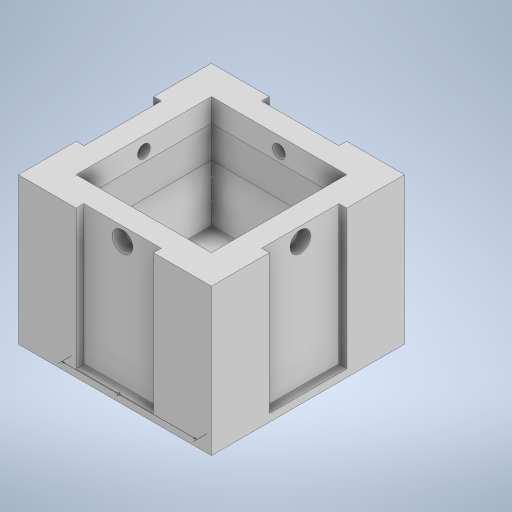
# Autodesk Inventor part: Ulepszona wersja
Saved by Autodesk Inventor 2024 (Build 280153000, 153)
## iProperties
Created: 2023-11-08
Part Number: Ulepszona wersja
Material: Generic
Document SubType Name: Modeling
Designer: Piotrek
Density: 1 g/cm^3
Appearance: Default
Author: Piotrek
Autodesk Inventor part; units mm, degrees
ref_plane "YZ Plane" through (0, 0, 0) normal (1, 0, 0) x (0, 1, 0)
ref_plane "XZ Plane" through (0, 0, 0) normal (0, 1, 0) x (-1, 0, 0)
sketch "Sketch1" plane through (0, 0, 0) normal (0, 1, 0) x (-1, 0, 0)
  line L0 (25, 25) -> (-25, 25)
  line L1 (-25, 25) -> (-25, -25)
  line L2 (-25, -25) -> (25, -25)
  line L3 (25, -25) -> (25, 25)
  line L4 (25, 25) -> (-25, -25) construction
  line L5 (-25, 25) -> (25, -25) construction
  line L6 (-22.5, 22.5) -> (22.5, 22.5)
  line L7 (22.5, 22.5) -> (22.5, -22.5)
  line L8 (22.5, -22.5) -> (-22.5, -22.5)
  line L9 (-22.5, -22.5) -> (-22.5, 22.5)
  line L10 (-22.5, 22.5) -> (22.5, -22.5) construction
  line L11 (22.5, 22.5) -> (-22.5, -22.5) construction
  point P0 (0, 0)
  dimension "d0" = 50
  dimension "d1" = 50
  dimension "d2" = 45
  dimension "d3" = 45
  constraints: 24 end point, 4 midpoint, 4 parallel, 2 horizontal, 2 perpendicular
  measures "d0" distance of L2.end L1.end
  measures "d1" distance of L1.end L0.end
  measures "d2" distance of L7.end L8.end
  measures "d3" distance of L6.end L7.end
extrude "Extrusion1" add sketch "Sketch1" along normal blind 30
extrude "Extrusion2" add sketch "Sketch1" along normal blind 2 contours L6 L7 L8 L9
sketch "Sketch2" plane through (0, 30, 0) normal (0, 1, 0) x (1, 0, 0)
  point P0 (0, 0)
sketch "Sketch3" plane through (0, 30, 0) normal (0, 1, 0) x (1, 0, 0)
  line L0 (17.5, -17.5) -> (-17.5, -17.5)
  line L1 (-17.5, -17.5) -> (-17.5, 17.5)
  line L2 (-17.5, 17.5) -> (17.5, 17.5)
  line L3 (17.5, 17.5) -> (17.5, -17.5)
  line L4 (17.5, -17.5) -> (-17.5, 17.5) construction
  line L5 (-17.5, -17.5) -> (17.5, 17.5) construction
  line L6 (-25, 25) -> (-25, -25) projected
  line L7 (25, -25) -> (-25, -25)
  line L8 (-25, -25) -> (-25, 25)
  line L9 (-25, 25) -> (25, 25)
  line L10 (25, 25) -> (25, -25)
  line L11 (25, -25) -> (-25, 25) construction
  line L12 (-25, -25) -> (25, 25) construction
  point P0 (0, 0)
  dimension "d8" = 35
  dimension "d9" = 35
  constraints: 24 end point, 4 midpoint, 4 parallel, 2 horizontal, 2 perpendicular
  measures "d8" distance of L1.end L2.end
  measures "d9" distance of L0.end L1.end
extrude "Extrusion3" add sketch "Sketch3" along normal blind 5.5
ref_plane "Work Plane1" through (0, 17.75, 0) normal (0, 1, 0) x (1, 0, 0)
chamfer "Chamfer1" distance 5 distance2 13.25 4 edges at (22.5, 30, 0) (0, 30, -22.5) (-22.5, 30, 0) (0, 30, 22.5) measured on face at (-5.8333, 30, 20.8333)
sketch "Sketch5" plane through (0, 35.5, 0) normal (0, 1, 0) x (1, 0, 0)
  point P0 (0, 0)
sketch "Sketch6" plane through (-17.5, 35.5, -17.5) normal (0, 0, 1) x (1, 0, 0)
  circle A0 centre (17.5, -3) radius 1.5
  line L0 (0, 0) -> (35, 0) projected
  point P0 (17.5, -35.5)
  point P1 (17.5, 0)
  dimension "d21" = 3
  dimension "d30" = 3
  constraints: 1 centre point, 1 midpoint
  measures "d21" diameter of A0
  measures "d30" distance of A0.centre point (17.5, 0)
extrude "Extrusion5" cut sketch "Sketch6" against normal through all
sketch "Sketch7" plane through (0, 35.5, 0) normal (0, 1, 0) x (1, 0, 0)
  line L0 (25, 25) -> (-25, 25) projected
  line L1 (10, 25) -> (0, 25)
  line L2 (10, 25) -> (-10, 25)
  line L3 (-10, 25) -> (10, 25)
  line L4 (10, 25) -> (10, 23)
  line L5 (10, 23) -> (-10, 23)
  line L6 (-10, 23) -> (-10, 25)
  point P0 (0, 0)
  dimension "d24" = 20
  dimension "d25" = 2
  constraints: 12 end point, 2 parallel, 2 point on line, 1 horizontal, 1 midpoint, 1 perpendicular
  measures "d24" distance of L1.start L2.end
  measures "d25" distance of L3.end L4.end
extrude "Extrusion6" cut sketch "Sketch7" against normal through all
sketch "Sketch9" plane through (10, 35.5, -23) normal (0, 0, -1) x (-1, 0, 0)
  circle A0 centre (10, -3) radius 1.5 projected
  circle A1 centre (10, -3) radius 2.5
  point P0 (10, -35.5)
  dimension "d37" = 3
  constraints: 1 centre point, 1 coincident
  measures "d37" diameter of A0
extrude "Extrusion7" cut sketch "Sketch9" against normal blind 3
pattern_circular "Circular Pattern2" count 4 over 360 about axis through (0, -10, 0) along (0, 1, 0) of "Extrusion7", "Extrusion6", "Extrusion5"
sketch "Sketch11" plane through (0, 32.5, -20) normal (0, 0, -1) x (-1, 0, 0)
  circle A0 centre (0, 0) radius 1.65
  circle A1 centre (0, 0) radius 2.65
  point P0 (0, -32.5)
  dimension "d38" = 3.3
  dimension "d39" = 5.3
  constraints: 2 centre point, 1 coincident
  measures "d38" diameter of A0
  measures "d39" diameter of A1
extrude "Extrusion9" cut sketch "Sketch11" against normal through all contours A0
extrude "Extrusion10" cut sketch "Sketch11" along normal blind 4
sketch "Sketch12" plane through (0, 32.5, 20) normal (0, 0, 1) x (1, 0, 0)
  circle A0 centre (0, 0) radius 2.65
  point P0 (0, -32.5)
  dimension "d44" = 5.3
  constraints: 1 centre point
  measures "d44" diameter of A0
extrude "Extrusion11" cut sketch "Sketch12" along normal blind 9
sketch "Sketch13" plane through (-20, 32.5, 0) normal (-1, 0, 0) x (0, 0, 1)
  circle A0 centre (0, 0) radius 1.65
  circle A1 centre (0, 0) radius 2.65
  point P0 (0, -32.5)
  dimension "d47" = 3.3
  dimension "d48" = 5.3
  constraints: 2 centre point, 1 coincident
  measures "d47" diameter of A0
  measures "d48" diameter of A1
extrude "Extrusion12" cut sketch "Sketch13" against normal through all contours A0
extrude "Extrusion13" cut sketch "Sketch13" along normal blind 9 contours A0 | A1
sketch "Sketch14" plane through (20, 32.5, 0) normal (1, 0, 0) x (0, 0, -1)
  circle A0 centre (0, 0) radius 2.65
  point P0 (0, -32.5)
  dimension "d53" = 5.3
  constraints: 1 centre point
  measures "d53" diameter of A0
extrude "Extrusion14" cut sketch "Sketch14" along normal blind 8.5
sketch "Sketch15" plane through (0, 35.5, 0) normal (0, 1, 0) x (1, 0, 0)
  line L0 (17.5, 17.5) -> (17.5, -17.5) projected
  line L1 (17.5, -17.5) -> (17.5, 17.5)
  line L2 (17.5, 17.5) -> (-17.5, 17.5)
  line L3 (-17.5, 17.5) -> (-17.5, -17.5)
  line L4 (-17.5, -17.5) -> (17.5, -17.5)
  line L5 (10, -23) -> (-10, -23) projected
  line L6 (10, -23) -> (10, -25)
  line L7 (10, -25) -> (25, -25)
  line L8 (25, -25) -> (25, -10)
  line L9 (23, -10) -> (23, 10) projected
  line L10 (25, -10) -> (23, -10)
  line L11 (23, -10) -> (23, 10)
  line L12 (23, 10) -> (25, 10)
  line L13 (25, 25) -> (10, 25) projected
  line L14 (25, 10) -> (25, 25)
  line L15 (25, 25) -> (10, 25)
  line L16 (10, 23) -> (-10, 23) projected
  line L17 (10, 25) -> (10, 23)
  line L18 (10, 23) -> (-10, 23)
  line L19 (-10, 23) -> (-10, 25)
  line L20 (-10, 25) -> (-25, 25) projected
  line L21 (-10, 25) -> (-25, 25)
  line L22 (-25, 25) -> (-25, 10)
  line L23 (-23, 10) -> (-23, -10) projected
  line L24 (-25, 10) -> (-23, 10)
  line L25 (-23, 10) -> (-23, -10)
  line L26 (-23, -10) -> (-25, -10)
  line L27 (-25, -10) -> (-25, -25)
  line L28 (-10, -23) -> (10, -23)
  line L29 (-10, -25) -> (-10, -23) projected
  line L30 (-10, -23) -> (-10, -25)
  line L31 (-10, -25) -> (-25, -25)
  point P0 (0, 0)
  dimension "d56" = 15
  dimension "d57" = 15
  constraints: 48 end point, 13 perpendicular, 8 point on line, 2 collinear, 1 vertical
  measures "d56" distance of L6.end L7.end
  measures "d57" distance of L7.end L8.end
extrude "Extrusion15" add sketch "Sketch15" along normal blind 0.5
extrude "Extrusion16" add sketch "Sketch1" against normal blind 2 contours L3 L2 L1 L0 | L6 L7 L8 L9
sketch "Sketch16" plane through (0, -2, 0) normal (0, -1, 0) x (1, 0, 0)
  line L0 (-15.5086, 20.4473) -> (19.4914, 20.4473) construction
  line L1 (19.4914, 20.4473) -> (19.4914, -17.6327) construction
  line L2 (19.4914, -17.6327) -> (-15.5086, -17.6327) construction
  line L3 (-15.5086, -17.6327) -> (-15.5086, 20.4473) construction
  point P0 (0, 0)
  dimension "d73" = 35
  constraints: 2 other
  measures "d73" distance of L0.start L0.end
body "Solid1"
